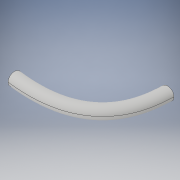
# Autodesk Inventor part: Wire to Power
Saved by Autodesk Inventor 2018 (Build 220112000, 112)
## iProperties
Created: 2018-07-20
Part Number: Wire to Power
Material: Generic
Document SubType Name: Modeling
Designer: DPLXuser
Density: 1 g/cm^3
Appearance: Default
Author: DPLXuser
Autodesk Inventor part; units mm, degrees
ref_plane "YZ Plane" through (0, 0, 0) normal (1, 0, 0) x (0, 1, 0)
ref_plane "XZ Plane" through (0, 0, 0) normal (0, 1, 0) x (-1, 0, 0)
ref_plane "XY Plane" through (0, 0, 0) normal (0, 0, 1) x (1, 0, 0)
sketch "Sketch1" plane through (0, 0, 0) normal (0, 1, 0) x (-1, 0, 0)
  line L0 (0, 0) -> (1.2573, 15.432) construction
  line L1 (1.2573, 15.432) -> (0, 74.7422) construction
  line L2 (0, 74.7422) -> (88.4627, 63.2535) construction
  spline S0 degree 3 poles (0, 0) (1.2573, 15.432) (0, 74.7422) (88.4627, 63.2535) knots 1 1 1 1 2 2 2 2
  constraints: 3 other
sketch "Sketch2" plane through (0, 0, 0) normal (0, 0, 1) x (1, 0, 0)
  circle A0 centre (0, 0) radius 6.35
  dimension "d0" = 12.7
  constraints: 1 centre point, 1 coincident
  measures "d0" diameter of A0
sweep "Sweep1" add profiles "Sketch2" path "Sketch1"
sketch "Sketch5" plane through (-88.4627, 0, 63.2535) normal (-0.9988551, 0, -0.0478374) x (-0.0478374, 0, 0.9988551)
  line L0 (-2.4654, 5.3462) -> (1.1205, 5.3462) construction
  line L1 (1.1205, 5.3462) -> (1.1205, -7.4556) construction
  line L2 (1.1205, -7.4556) -> (-2.4654, -7.4556) construction
  line L3 (-2.4654, -7.4556) -> (-2.4654, 5.3462) construction
  line L4 (-0.9389, 4.5657) -> (-1.2279, 2.2785)
  line L5 (-1.2279, 2.2785) -> (-1.4082, 2.2785)
  line L6 (-1.4082, 2.2785) -> (-1.6873, 4.0421)
  line L7 (-1.6873, 4.0421) -> (-1.964, 2.2785)
  line L8 (-1.964, 2.2785) -> (-2.1418, 2.2785)
  line L9 (-2.1418, 2.2785) -> (-2.4357, 4.5657)
  line L10 (-2.4357, 4.5657) -> (-2.2357, 4.5657)
  line L11 (-2.2357, 4.5657) -> (-2.0331, 2.7947)
  line L12 (-2.0331, 2.7947) -> (-1.7614, 4.5657)
  line L13 (-1.7614, 4.5657) -> (-1.6033, 4.5657)
  line L14 (-1.6033, 4.5657) -> (-1.3242, 2.7947)
  line L15 (-1.3242, 2.7947) -> (-1.134, 4.5657)
  line L16 (-1.134, 4.5657) -> (-0.9389, 4.5657)
  line L17 (-0.5733, 2.2785) -> (-0.766, 2.2785)
  line L18 (-0.766, 2.2785) -> (-0.766, 4.5657)
  line L19 (-0.766, 4.5657) -> (-0.5733, 4.5657)
  line L20 (-0.5733, 4.5657) -> (-0.5733, 2.2785)
  line L21 (-0.5585, 4.9461) -> (-0.7783, 4.9461)
  line L22 (-0.7783, 4.9461) -> (-0.7783, 5.3462)
  line L23 (-0.7783, 5.3462) -> (-0.5585, 5.3462)
  line L24 (-0.5585, 5.3462) -> (-0.5585, 4.9461)
  line L25 (0.3159, 4.1532) -> (0.306, 4.1532)
  spline S0 degree 2 poles (0.306, 4.1532) (0.2838, 4.1656) (0.2368, 4.1705) (0.2023, 4.1705) knots 0 0 0 1 2 2 2
  spline S1 degree 2 poles (0.2023, 4.1705) (0.1232, 4.1705) (-0.0299, 4.0347) (-0.0991, 3.9013) knots 0 0 0 1 2 2 2
  line L26 (-0.0991, 3.9013) -> (-0.0991, 2.2785)
  line L27 (-0.0991, 2.2785) -> (-0.2918, 2.2785)
  line L28 (-0.2918, 2.2785) -> (-0.2918, 4.5657)
  line L29 (-0.2918, 4.5657) -> (-0.0991, 4.5657)
  line L30 (-0.0991, 4.5657) -> (-0.0991, 4.2249)
  spline S2 degree 2 poles (-0.0991, 4.2249) (0.0071, 4.4126) (0.1627, 4.5657) (0.2368, 4.5657) knots 0 0 0 1 2 2 2
  spline S3 degree 2 poles (0.2368, 4.5657) (0.2665, 4.5657) (0.2986, 4.5608) (0.3159, 4.5534) knots 0 0 0 1 2 2 2
  line L31 (0.3159, 4.5534) -> (0.3159, 4.1532)
  spline S4 degree 2 poles (0.9581, 2.2266) (0.6864, 2.2266) (0.385, 2.8416) (0.385, 3.4098) knots 0 0 0 1 2 2 2
  spline S5 degree 2 poles (0.385, 3.4098) (0.385, 3.968) (0.6765, 4.6299) (0.9136, 4.6299) knots 0 0 0 1 2 2 2
  spline S6 degree 2 poles (0.9136, 4.6299) (1.0198, 4.6299) (1.1828, 4.5064) (1.2446, 4.3755) knots 0 0 0 1 2 2 2
  spline S7 degree 2 poles (1.2446, 4.3755) (1.3063, 4.2446) (1.3706, 3.8667) (1.3706, 3.5925) knots 0 0 0 1 2 2 2
  line L32 (1.3706, 3.5925) -> (1.3706, 3.3826)
  line L33 (1.3706, 3.3826) -> (0.5777, 3.3826)
  spline S8 degree 2 poles (0.5777, 3.3826) (0.5777, 2.9849) (0.7778, 2.5625) (0.9556, 2.5625) knots 0 0 0 1 2 2 2
  spline S9 degree 2 poles (0.9556, 2.5625) (1.0198, 2.5625) (1.1409, 2.6193) (1.1903, 2.6638) knots 0 0 0 1 2 2 2
  spline S10 degree 2 poles (1.1903, 2.6638) (1.2421, 2.7132) (1.3138, 2.7997) (1.336, 2.8392) knots 0 0 0 1 2 2 2
  line L34 (1.336, 2.8392) -> (1.3483, 2.8392)
  line L35 (1.3483, 2.8392) -> (1.3483, 2.4193)
  spline S11 degree 2 poles (1.3483, 2.4193) (1.3138, 2.3921) (1.215, 2.3131) (1.1754, 2.2908) knots 0 0 0 1 2 2 2
  spline S12 degree 2 poles (1.1754, 2.2908) (1.1186, 2.2587) (1.0272, 2.2266) (0.9581, 2.2266) knots 0 0 0 1 2 2 2
  spline S13 degree 2 poles (1.1828, 3.6765) (1.1804, 3.8321) (1.1483, 4.0594) (1.1162, 4.1359) knots 0 0 0 1 2 2 2
  spline S14 degree 2 poles (1.1162, 4.1359) (1.084, 4.2224) (0.9778, 4.3138) (0.9013, 4.3138) knots 0 0 0 1 2 2 2
  spline S15 degree 2 poles (0.9013, 4.3138) (0.8247, 4.3138) (0.716, 4.2224) (0.6716, 4.1335) knots 0 0 0 1 2 2 2
  spline S16 degree 2 poles (0.6716, 4.1335) (0.6296, 4.0421) (0.5826, 3.8222) (0.5777, 3.6765) knots 0 0 0 1 2 2 2
  line L36 (0.5777, 3.6765) -> (1.1828, 3.6765)
  spline S17 degree 2 poles (-1.9788, -0.814) (-2.1369, -0.814) (-2.3147, -0.4558) (-2.3147, -0.068) knots 0 0 0 1 2 2 2
  line L37 (-2.3147, -0.068) -> (-2.3147, 1.1991)
  line L38 (-2.3147, 1.1991) -> (-2.4456, 1.1991)
  line L39 (-2.4456, 1.1991) -> (-2.4456, 1.5177)
  line L40 (-2.4456, 1.5177) -> (-2.3147, 1.5177)
  line L41 (-2.3147, 1.5177) -> (-2.3147, 2.1747)
  line L42 (-2.3147, 2.1747) -> (-2.122, 2.1747)
  line L43 (-2.122, 2.1747) -> (-2.122, 1.5177)
  line L44 (-2.122, 1.5177) -> (-1.7664, 1.5177)
  line L45 (-1.7664, 1.5177) -> (-1.7664, 1.1991)
  line L46 (-1.7664, 1.1991) -> (-2.122, 1.1991)
  line L47 (-2.122, 1.1991) -> (-2.122, 0.1098)
  spline S18 degree 2 poles (-2.122, 0.1098) (-2.122, -0.0631) (-2.1146, -0.2533) (-2.0949, -0.3348) knots 0 0 0 1 2 2 2
  spline S19 degree 2 poles (-2.0949, -0.3348) (-2.0776, -0.4064) (-1.9985, -0.4781) (-1.9318, -0.4781) knots 0 0 0 1 2 2 2
  spline S20 degree 2 poles (-1.9318, -0.4781) (-1.8849, -0.4781) (-1.796, -0.4212) (-1.7787, -0.404) knots 0 0 0 1 2 2 2
  line L48 (-1.7787, -0.404) -> (-1.7664, -0.404)
  line L49 (-1.7664, -0.404) -> (-1.7664, -0.7498)
  spline S21 degree 2 poles (-1.7664, -0.7498) (-1.8207, -0.7794) (-1.9318, -0.814) (-1.9788, -0.814) knots 0 0 0 1 2 2 2
  spline S22 degree 2 poles (-0.6845, 0.3741) (-0.6845, -0.2039) (-0.9636, -0.8337) (-1.1933, -0.8337) knots 0 0 0 1 2 2 2
  spline S23 degree 2 poles (-1.1933, -0.8337) (-1.4329, -0.8337) (-1.7046, -0.1841) (-1.7046, 0.3741) knots 0 0 0 1 2 2 2
  spline S24 degree 2 poles (-1.7046, 0.3741) (-1.7046, 0.9471) (-1.423, 1.5819) (-1.1933, 1.5819) knots 0 0 0 1 2 2 2
  spline S25 degree 2 poles (-1.1933, 1.5819) (-0.9636, 1.5819) (-0.6845, 0.9496) (-0.6845, 0.3741) knots 0 0 0 1 2 2 2
  spline S26 degree 2 poles (-0.8821, 0.3741) (-0.8821, 0.8187) (-1.0451, 1.251) (-1.1933, 1.251) knots 0 0 0 1 2 2 2
  spline S27 degree 2 poles (-1.1933, 1.251) (-1.344, 1.251) (-1.507, 0.8187) (-1.507, 0.3741) knots 0 0 0 1 2 2 2
  spline S28 degree 2 poles (-1.507, 0.3741) (-1.507, -0.0581) (-1.344, -0.5028) (-1.1933, -0.5028) knots 0 0 0 1 2 2 2
  spline S29 degree 2 poles (-1.1933, -0.5028) (-1.0451, -0.5028) (-0.8821, -0.0656) (-0.8821, 0.3741) knots 0 0 0 1 2 2 2
  spline S30 degree 2 poles (-1.3662, -2.6368) (-1.3662, -3.1975) (-1.6379, -3.8817) (-1.8429, -3.8817) knots 0 0 0 1 2 2 2
  spline S31 degree 2 poles (-1.8429, -3.8817) (-1.9368, -3.8817) (-2.0702, -3.7903) (-2.1344, -3.7113) knots 0 0 0 1 2 2 2
  line L50 (-2.1344, -3.7113) -> (-2.1467, -3.8175)
  line L51 (-2.1467, -3.8175) -> (-2.327, -3.8175)
  line L52 (-2.327, -3.8175) -> (-2.327, -0.6337)
  line L53 (-2.327, -0.6337) -> (-2.1344, -0.6337)
  line L54 (-2.1344, -0.6337) -> (-2.1344, -1.7699)
  spline S32 degree 2 poles (-2.1344, -1.7699) (-2.0628, -1.639) (-1.8923, -1.4661) (-1.7836, -1.4661) knots 0 0 0 1 2 2 2
  spline S33 degree 2 poles (-1.7836, -1.4661) (-1.591, -1.4661) (-1.3662, -2.086) (-1.3662, -2.6368) knots 0 0 0 1 2 2 2
  spline S34 degree 2 poles (-1.5638, -2.6665) (-1.5638, -2.2565) (-1.6898, -1.8316) (-1.8281, -1.8316) knots 0 0 0 1 2 2 2
  spline S35 degree 2 poles (-1.8281, -1.8316) (-1.9071, -1.8316) (-2.0677, -1.9798) (-2.1344, -2.0934) knots 0 0 0 1 2 2 2
  line L55 (-2.1344, -2.0934) -> (-2.1344, -3.405)
  spline S36 degree 2 poles (-2.1344, -3.405) (-2.0603, -3.4767) (-1.9491, -3.5359) (-1.88, -3.5359) knots 0 0 0 1 2 2 2
  spline S37 degree 2 poles (-1.88, -3.5359) (-1.7318, -3.5359) (-1.5638, -3.1185) (-1.5638, -2.6665) knots 0 0 0 1 2 2 2
  spline S38 degree 2 poles (-0.5289, -3.5755) (-0.5536, -3.61) (-0.6301, -3.7335) (-0.6672, -3.7706) knots 0 0 0 1 2 2 2
  spline S39 degree 2 poles (-0.6672, -3.7706) (-0.7191, -3.8249) (-0.8154, -3.8817) (-0.8994, -3.8817) knots 0 0 0 1 2 2 2
  spline S40 degree 2 poles (-0.8994, -3.8817) (-0.971, -3.8817) (-1.097, -3.7755) (-1.1464, -3.6792) knots 0 0 0 1 2 2 2
  spline S41 degree 2 poles (-1.1464, -3.6792) (-1.1933, -3.5853) (-1.2476, -3.3087) (-1.2476, -3.1556) knots 0 0 0 1 2 2 2
  spline S42 degree 2 poles (-1.2476, -3.1556) (-1.2476, -2.9184) (-1.1464, -2.5825) (-1.0377, -2.4862) knots 0 0 0 1 2 2 2
  spline S43 degree 2 poles (-1.0377, -2.4862) (-0.9414, -2.3973) (-0.6795, -2.3306) (-0.5289, -2.3133) knots 0 0 0 1 2 2 2
  line L56 (-0.5289, -2.3133) -> (-0.5289, -2.2392)
  spline S44 degree 2 poles (-0.5289, -2.2392) (-0.5289, -2.1058) (-0.5709, -1.9403) (-0.6054, -1.8934) knots 0 0 0 1 2 2 2
  spline S45 degree 2 poles (-0.6054, -1.8934) (-0.6425, -1.8464) (-0.7487, -1.8168) (-0.8055, -1.8168) knots 0 0 0 1 2 2 2
  spline S46 degree 2 poles (-0.8055, -1.8168) (-0.8722, -1.8168) (-1.0525, -1.8958) (-1.1414, -1.9724) knots 0 0 0 1 2 2 2
  line L57 (-1.1414, -1.9724) -> (-1.1538, -1.9724)
  line L58 (-1.1538, -1.9724) -> (-1.1538, -1.5797)
  spline S47 degree 2 poles (-1.1538, -1.5797) (-1.0994, -1.55) (-0.9018, -1.4759) (-0.8055, -1.4759) knots 0 0 0 1 2 2 2
  spline S48 degree 2 poles (-0.8055, -1.4759) (-0.687, -1.4759) (-0.5239, -1.55) (-0.4597, -1.6464) knots 0 0 0 1 2 2 2
  spline S49 degree 2 poles (-0.4597, -1.6464) (-0.398, -1.7402) (-0.3362, -2.0391) (-0.3362, -2.254) knots 0 0 0 1 2 2 2
  line L59 (-0.3362, -2.254) -> (-0.3362, -3.8175)
  line L60 (-0.3362, -3.8175) -> (-0.5289, -3.8175)
  line L61 (-0.5289, -3.8175) -> (-0.5289, -3.5755)
  line L62 (-0.5289, -3.2544) -> (-0.5289, -2.6196)
  spline S50 degree 2 poles (-0.5289, -2.6196) (-0.598, -2.6319) (-0.808, -2.6739) (-0.8722, -2.7134) knots 0 0 0 1 2 2 2
  spline S51 degree 2 poles (-0.8722, -2.7134) (-0.9488, -2.7603) (-1.05, -2.9555) (-1.05, -3.1284) knots 0 0 0 1 2 2 2
  spline S52 degree 2 poles (-1.05, -3.1284) (-1.05, -3.326) (-0.9389, -3.5261) (-0.8327, -3.5261) knots 0 0 0 1 2 2 2
  spline S53 degree 2 poles (-0.8327, -3.5261) (-0.7413, -3.5261) (-0.5931, -3.3704) (-0.5289, -3.2544) knots 0 0 0 1 2 2 2
  spline S54 degree 2 poles (0.2788, -3.862) (0.1207, -3.862) (-0.0571, -3.5038) (-0.0571, -3.116) knots 0 0 0 1 2 2 2
  line L63 (-0.0571, -3.116) -> (-0.0571, -1.8489)
  line L64 (-0.0571, -1.8489) -> (-0.188, -1.8489)
  line L65 (-0.188, -1.8489) -> (-0.188, -1.5303)
  line L66 (-0.188, -1.5303) -> (-0.0571, -1.5303)
  line L67 (-0.0571, -1.5303) -> (-0.0571, -0.8733)
  line L68 (-0.0571, -0.8733) -> (0.1356, -0.8733)
  line L69 (0.1356, -0.8733) -> (0.1356, -1.5303)
  line L70 (0.1356, -1.5303) -> (0.4912, -1.5303)
  line L71 (0.4912, -1.5303) -> (0.4912, -1.8489)
  line L72 (0.4912, -1.8489) -> (0.1356, -1.8489)
  line L73 (0.1356, -1.8489) -> (0.1356, -2.9382)
  spline S55 degree 2 poles (0.1356, -2.9382) (0.1356, -3.1111) (0.143, -3.3013) (0.1627, -3.3828) knots 0 0 0 1 2 2 2
  spline S56 degree 2 poles (0.1627, -3.3828) (0.18, -3.4544) (0.2591, -3.5261) (0.3258, -3.5261) knots 0 0 0 1 2 2 2
  spline S57 degree 2 poles (0.3258, -3.5261) (0.3727, -3.5261) (0.4616, -3.4692) (0.4789, -3.452) knots 0 0 0 1 2 2 2
  line L74 (0.4789, -3.452) -> (0.4912, -3.452)
  line L75 (0.4912, -3.452) -> (0.4912, -3.7978)
  spline S58 degree 2 poles (0.4912, -3.7978) (0.4369, -3.8274) (0.3258, -3.862) (0.2788, -3.862) knots 0 0 0 1 2 2 2
  spline S59 degree 2 poles (0.9803, -3.862) (0.8222, -3.862) (0.6444, -3.5038) (0.6444, -3.116) knots 0 0 0 1 2 2 2
  line L76 (0.6444, -3.116) -> (0.6444, -1.8489)
  line L77 (0.6444, -1.8489) -> (0.5135, -1.8489)
  line L78 (0.5135, -1.8489) -> (0.5135, -1.5303)
  line L79 (0.5135, -1.5303) -> (0.6444, -1.5303)
  line L80 (0.6444, -1.5303) -> (0.6444, -0.8733)
  line L81 (0.6444, -0.8733) -> (0.837, -0.8733)
  line L82 (0.837, -0.8733) -> (0.837, -1.5303)
  line L83 (0.837, -1.5303) -> (1.1927, -1.5303)
  line L84 (1.1927, -1.5303) -> (1.1927, -1.8489)
  line L85 (1.1927, -1.8489) -> (0.837, -1.8489)
  line L86 (0.837, -1.8489) -> (0.837, -2.9382)
  spline S60 degree 2 poles (0.837, -2.9382) (0.837, -3.1111) (0.8445, -3.3013) (0.8642, -3.3828) knots 0 0 0 1 2 2 2
  spline S61 degree 2 poles (0.8642, -3.3828) (0.8815, -3.4544) (0.9605, -3.5261) (1.0272, -3.5261) knots 0 0 0 1 2 2 2
  spline S62 degree 2 poles (1.0272, -3.5261) (1.0742, -3.5261) (1.1631, -3.4692) (1.1804, -3.452) knots 0 0 0 1 2 2 2
  line L87 (1.1804, -3.452) -> (1.1927, -3.452)
  line L88 (1.1927, -3.452) -> (1.1927, -3.7978)
  spline S63 degree 2 poles (1.1927, -3.7978) (1.1384, -3.8274) (1.0272, -3.862) (0.9803, -3.862) knots 0 0 0 1 2 2 2
  spline S64 degree 2 poles (1.8275, -3.8694) (1.5558, -3.8694) (1.2545, -3.2544) (1.2545, -2.6862) knots 0 0 0 1 2 2 2
  spline S65 degree 2 poles (1.2545, -2.6862) (1.2545, -2.128) (1.5459, -1.4661) (1.7831, -1.4661) knots 0 0 0 1 2 2 2
  spline S66 degree 2 poles (1.7831, -1.4661) (1.8893, -1.4661) (2.0523, -1.5896) (2.114, -1.7205) knots 0 0 0 1 2 2 2
  spline S67 degree 2 poles (2.114, -1.7205) (2.1758, -1.8514) (2.24, -2.2293) (2.24, -2.5035) knots 0 0 0 1 2 2 2
  line L89 (2.24, -2.5035) -> (2.24, -2.7134)
  line L90 (2.24, -2.7134) -> (1.4471, -2.7134)
  spline S68 degree 2 poles (1.4471, -2.7134) (1.4471, -3.1111) (1.6472, -3.5335) (1.8251, -3.5335) knots 0 0 0 1 2 2 2
  spline S69 degree 2 poles (1.8251, -3.5335) (1.8893, -3.5335) (2.0103, -3.4767) (2.0597, -3.4322) knots 0 0 0 1 2 2 2
  spline S70 degree 2 poles (2.0597, -3.4322) (2.1116, -3.3828) (2.1832, -3.2963) (2.2054, -3.2568) knots 0 0 0 1 2 2 2
  line L91 (2.2054, -3.2568) -> (2.2178, -3.2568)
  line L92 (2.2178, -3.2568) -> (2.2178, -3.6767)
  spline S71 degree 2 poles (2.2178, -3.6767) (2.1832, -3.7039) (2.0844, -3.7829) (2.0449, -3.8052) knots 0 0 0 1 2 2 2
  spline S72 degree 2 poles (2.0449, -3.8052) (1.9881, -3.8373) (1.8967, -3.8694) (1.8275, -3.8694) knots 0 0 0 1 2 2 2
  spline S73 degree 2 poles (2.0523, -2.4195) (2.0498, -2.2639) (2.0177, -2.0366) (1.9856, -1.9601) knots 0 0 0 1 2 2 2
  spline S74 degree 2 poles (1.9856, -1.9601) (1.9535, -1.8736) (1.8473, -1.7822) (1.7707, -1.7822) knots 0 0 0 1 2 2 2
  spline S75 degree 2 poles (1.7707, -1.7822) (1.6941, -1.7822) (1.5855, -1.8736) (1.541, -1.9625) knots 0 0 0 1 2 2 2
  spline S76 degree 2 poles (1.541, -1.9625) (1.499, -2.0539) (1.4521, -2.2738) (1.4471, -2.4195) knots 0 0 0 1 2 2 2
  line L93 (1.4471, -2.4195) -> (2.0523, -2.4195)
  line L94 (3.0452, -1.9428) -> (3.0354, -1.9428)
  spline S77 degree 2 poles (3.0354, -1.9428) (3.0131, -1.9304) (2.9662, -1.9255) (2.9316, -1.9255) knots 0 0 0 1 2 2 2
  spline S78 degree 2 poles (2.9316, -1.9255) (2.8526, -1.9255) (2.6994, -2.0613) (2.6303, -2.1947) knots 0 0 0 1 2 2 2
  line L95 (2.6303, -2.1947) -> (2.6303, -3.8175)
  line L96 (2.6303, -3.8175) -> (2.4376, -3.8175)
  line L97 (2.4376, -3.8175) -> (2.4376, -1.5303)
  line L98 (2.4376, -1.5303) -> (2.6303, -1.5303)
  line L99 (2.6303, -1.5303) -> (2.6303, -1.8711)
  spline S79 degree 2 poles (2.6303, -1.8711) (2.7365, -1.6834) (2.8921, -1.5303) (2.9662, -1.5303) knots 0 0 0 1 2 2 2
  spline S80 degree 2 poles (2.9662, -1.5303) (2.9958, -1.5303) (3.028, -1.5352) (3.0452, -1.5426) knots 0 0 0 1 2 2 2
  line L100 (3.0452, -1.5426) -> (3.0452, -1.9428)
  line L101 (4.095, -1.5303) -> (3.4775, -4.6598)
  line L102 (3.4775, -4.6598) -> (3.27, -4.6598)
  line L103 (3.27, -4.6598) -> (3.4775, -3.7064)
  line L104 (3.4775, -3.7064) -> (3.0601, -1.5303)
  line L105 (3.0601, -1.5303) -> (3.2675, -1.5303)
  line L106 (3.2675, -1.5303) -> (3.5812, -3.2272)
  line L107 (3.5812, -3.2272) -> (3.8925, -1.5303)
  line L108 (3.8925, -1.5303) -> (4.095, -1.5303)
  point P0 (-67.4129, 0)
  constraints: 2 other
emboss "Emboss1" sketch "Sketch5" operation add depth 0.254 direction (0.9988551, 0, 0.0478374)
body "Solid1"
